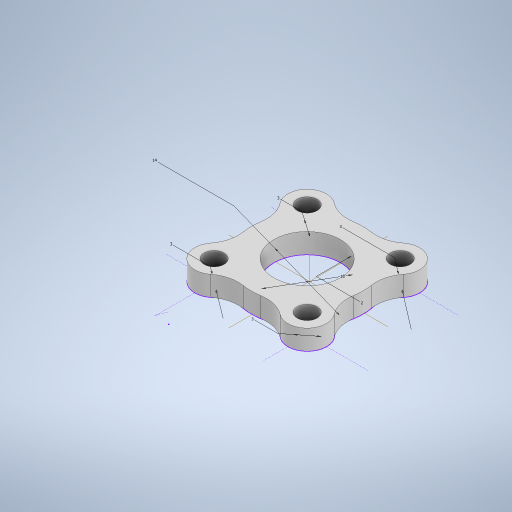
# Autodesk Inventor part: крепление подшипника_1_CPY
Saved by Autodesk Inventor 2024.2 (Build 282272000, 272)
## iProperties
Created: 2025-11-25
Part Number: крепление подшипника_1_CPY
Material: Типовые
Document SubType Name: Modeling
Designer: Service
Density: 1 g/cm^3
Appearance: По умолчанию
Author: Zakhar
Autodesk Inventor part; units mm, degrees
ref_plane "YZ Plane" through (0, 0, 0) normal (1, 0, 0) x (0, 1, 0)
ref_plane "XZ Plane" through (0, 0, 0) normal (0, 1, 0) x (-1, 0, 0)
ref_plane "XY Plane" through (0, 0, 0) normal (0, 0, 1) x (1, 0, 0)
sketch "Эскиз1" plane through (0, 0, 0) normal (0, 1, 0) x (-1, 0, 0)
  circle A0 centre (0.1295, 0.2019) radius 7
  circle A1 centre (-6.8705, 7.2019) radius 1.5
  circle A2 centre (7.1295, 7.2019) radius 1.5
  circle A3 centre (7.1295, -6.7981) radius 1.5
  circle A4 centre (-6.8705, -6.7981) radius 1.5
  line L0 (-6.8705, -10.8093) -> (-6.8705, 13.8282) construction
  line L1 (14.3213, 7.2019) -> (-16.097, 7.2019) construction
  line L2 (7.1295, -11.068) -> (7.1295, 16.1729) construction
  arc A5 (6.5047, 14.6631) -> (7.1295, 16.1729) centre (4.9928, 16.1729) ccw construction
  line L3 (12.5583, -6.7981) -> (-15.6188, -6.7981) construction
  circle A6 centre (7.1295, 7.2019) radius 2.8995
  circle A7 centre (-6.8705, 7.2019) radius 2.8995
  circle A8 centre (-6.8705, -6.7981) radius 2.8995
  circle A9 centre (7.1295, -6.7981) radius 2.8995
  arc A10 (0.5599, -6.4772) -> (-0.2768, -6.4772) centre (0.1416, -8.4329) ccw
  line L4 (5.6295, -6.7981) -> (0.1295, -6.7981)
  line L5 (7.1295, -5.2981) -> (7.1295, 0.2019)
  line L6 (7.1295, 5.7019) -> (7.1295, 0.2019)
  line L7 (5.6295, 7.2019) -> (-5.3705, 7.2019)
  line L8 (-6.8705, 5.7019) -> (-6.8705, -5.2981)
  line L9 (-5.3705, -6.7981) -> (0.1295, -6.7981)
  circle A11 centre (0.1295, 0.2019) radius 8.3995
  circle A12 centre (0.1295, 0.2019) radius 5
  point P0 (-3.971, 7.2019)
  point P1 (-6.8705, 4.3024)
  point P2 (-6.8705, -3.8986)
  point P3 (-3.971, -6.7981)
  point P4 (4.23, -6.7981)
  point P5 (7.1295, -3.8986)
  point P6 (7.1295, 4.3024)
  point P7 (4.23, 7.2019)
  point P8 (4.2478, 7.5225)
  point P9 (-3.9888, 7.5225)
  point P10 (-7.1911, 4.3202)
  point P11 (-7.1911, -3.9164)
  point P12 (-3.9888, -7.1187)
  point P13 (4.2478, -7.1187)
  point P14 (7.4501, -3.9164)
  point P15 (7.4501, 4.3202)
  dimension "d23" = 14
  dimension "d24" = 3
  dimension "d25" = 3
  dimension "d26" = 3
  dimension "d27" = 3
  dimension "d28" = 2
  dimension "d40" = 10
  constraints: 20 end point, 15 point on line, 14 point on circle, 13 centre point, 11 tangent, 6 coincident, 3 perpendicular, 1 collinear, 1 vertical
  measures "d23" diameter of A0
  measures "d24" diameter of A1
  measures "d25" diameter of A2
  measures "d26" diameter of A3
  measures "d27" diameter of A4
  measures "d28" radius of A10
  measures "d40" diameter of A12
extrude "Выдавливание1" add sketch "Эскиз1" along normal blind 3 contours L5 A9 A0 | L6 A6 A11 A9 L5 | A0 A6 L6 | A0 L7 A6 | A6 L7 A11 L6 | A9 L4 A0 | A9 L5 A11 L4 | A9 A11 L5 | L6 A11 A6 | L7 A7 A11 A6 | A0 A7 L7 | A6 A11 L7 | L9 A8 A0 | L4 A9 A11 A8 L9 | L4 A11 A9 | A9 A11 L4 A3 L5 | L5 A3 A11 | A11 L6 A2 L7 A6 | A11 A2 L6 | A0 L8 A7 | A7 L8 A11 L7 | L7 A11 A7 | L7 A2 A11 | A8 L8 A0 | A8 L9 A11 L8 | A8 A11 L9 | A11 A3 L4 | L8 A8 A11 A7 | A7 A11 L8 | A11 L7 A1 L8 A7 | A11 A1 L7 | L8 A11 A8 | A8 A11 L8 A4 L9 | L9 A4 A11 | L8 A1 A11 | A11 A4 L8
extrude "Выдавливание3" add sketch "Эскиз1" along normal up to surface (3 mm away) contours A0
fillet "Сопряжение грани1" radius 5 1 edges at (-4.2478, 1.5, 7.5225)
fillet "Сопряжение грани2" radius 5 1 edges at (3.9888, 1.5, 7.5225)
fillet "Сопряжение грани3" radius 5 1 edges at (7.1911, 1.5, 4.3202)
fillet "Сопряжение грани4" radius 5 1 edges at (7.1911, 1.5, -3.9164)
fillet "Сопряжение грани5" radius 5 1 edges at (-4.2478, 1.5, -7.1187)
fillet "Сопряжение грани6" radius 5 1 edges at (3.9888, 1.5, -7.1187)
fillet "Сопряжение грани7" radius 5 1 edges at (-7.4501, 1.5, -3.9164)
fillet "Сопряжение грани8" radius 5 1 edges at (-7.4501, 1.5, 4.3202)
